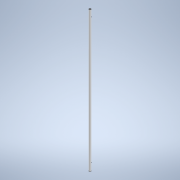
# Autodesk Inventor part: burder_rod_2
Saved by Autodesk Inventor 2020 (Build 240168000, 168)
## iProperties
Created: 2019-06-12
Part Number: burder_rod_2
Material: Generic
Document SubType Name: Modeling
Designer: ColinP
Density: 1 g/cm^3
Appearance: Default
Author: ColinP
Autodesk Inventor part; units mm, degrees
ref_plane "YZ Plane" through (0, 0, 0) normal (1, 0, 0) x (0, 1, 0)
ref_plane "XZ Plane" through (0, 0, 0) normal (0, 1, 0) x (-1, 0, 0)
ref_plane "XY Plane" through (0, 0, 0) normal (0, 0, 1) x (1, 0, 0)
sketch "Sketch1" plane through (0, 0, 0) normal (0, 1, 0) x (-1, 0, 0)
  circle A0 centre (0, 0) radius 1.5875
  dimension "d0" = 3.175
  constraints: 1 centre point, 1 coincident
  measures "d0" diameter of A0
extrude "Extrusion1" add sketch "Sketch1" along normal blind 254
sketch "Sketch2" plane through (0, 254, 0) normal (0, 1, 0) x (1, 0, 0)
  circle A0 centre (0, 0) radius 1.5875 projected
  constraints: 1 coincident
hole "Hole1" at (0, 254, 0) direction (0, -1, 0) diameter 2.159 end through all
sketch "Sketch3" plane through (0, 0, 0) normal (0, 0, 1) x (1, 0, 0)
  line L0 (1.5875, 0) -> (-1.5875, 0) projected
  line L1 (0, 0) -> (0, 6.35)
  line L2 (0, 0) -> (6.35, 0) construction
  line L3 (0, 6.35) -> (0, 8.89)
  line L4 (0, 8.89) -> (0, 12.7)
  line L5 (0, 8.89) -> (3.81, 8.89) construction
  circle A0 centre (0, 12.7) radius 0.635
  dimension "d10" = 6.35
  dimension "d11" = 270
  dimension "d12" = 2.54
  dimension "d13" = 3.81
  dimension "d14" = 90
  dimension "d15" = 1.27
  constraints: 10 end point, 2 horizontal, 2 perpendicular, 2 vertical, 1 centre point, 1 coincident, 1 point on line
  measures "d10" distance of L1.start L1.end
  measures "d12" distance of L1.end L3.end
  measures "d13" distance of L3.end L4.end
  measures "d14" angle of L5 L4
  measures "d15" diameter of A0
sketch "Sketch4" plane through (0, 0, 0) normal (0, 1, 0) x (-1, 0, 0)
  point P0 (0, 0)
sketch "Sketch5" plane through (0, 0, 0) normal (0, 0, 1) x (1, 0, 0)
  line L0 (-1.0795, 254) -> (1.0795, 254) projected
  line L1 (0, 254) -> (0, 241.3)
  circle A0 centre (0, 241.3) radius 0.635
  point P0 (0, 0)
  dimension "d16" = 12.7
  dimension "d17" = 1.27
  constraints: 2 end point, 1 centre point, 1 coincident, 1 midpoint, 1 vertical
  measures "d16" distance of L1.start L1.end
  measures "d17" diameter of A0
hole "Hole2" at (0, 241.3, 0) direction (0, 0, -1) diameter 1.27 depth 1.5875 tip angle 118
hole "Hole3" at (0, 12.7, 0) direction (0, 0, -1) diameter 1.27 depth 1.5875 tip angle 118
body "Solid1"
